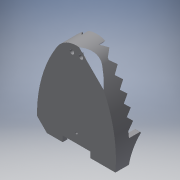
# Autodesk Inventor part: HeadFrame
Saved by Autodesk Inventor 2016 (Build 200138000, 138)
## iProperties
Created: 2017-03-13
Part Number: HeadFrame
Material: Generic
Document SubType Name: Modeling
Designer: Owner
Density: 1 g/cm^3
Appearance: Default
Author: Owner
Autodesk Inventor part; units mm, degrees
sketch "Sketch1" plane through (0, 0, 0) normal (0, 0, 1) x (1, 0, 0)
  line L0 (43.1, 62.15) -> (-43.1, 62.15) projected
  line L1 (43.1, 62.15) -> (-43.1, 62.15)
  line L2 (-43.1, 62.15) -> (-43.1, 176.45)
  line L3 (-43.1, 176.45) -> (43.1, 176.45)
  line L4 (43.1, 176.45) -> (43.1, 62.15)
  arc A0 (43.1, 62.15) -> (21.3882, 150.6616) centre (-96.2036, 74.8977) ccw
  arc A1 (-21.3307, 150.6382) -> (-43.1, 62.15) centre (96.939, 74.6204) ccw
  arc A2 (21.3882, 150.6616) -> (-21.3307, 150.6382) centre (0.0363, 136.9046) ccw
  point P0 (0, 0)
  dimension "d0" = 114.3
  dimension "d1" = 25.4
  constraints: 8 end point, 6 point on circle, 3 centre point, 2 parallel, 2 tangent, 1 horizontal, 1 perpendicular
  measures "d0" distance of L3.end L0.start
  measures "d1" radius of A2
extrude "Extrusion1" add sketch "Sketch1" against normal blind 5 contours L0 L2 A1 A2 A0 L4 | L4 A0 | A1 L2
sketch "Sketch2" plane through (0, 0, -5) normal (0, 0, -1) x (-1, 0, 0)
  arc A0 (-21.3882, 150.6616) -> (-43.1, 62.15) centre (96.2036, 74.8977) ccw projected
  line L0 (-43.1, 62.15) -> (43.1, 62.15) projected
  arc A1 (43.1, 62.15) -> (21.3307, 150.6382) centre (-96.939, 74.6204) ccw projected
  arc A2 (21.3307, 150.6382) -> (-21.3882, 150.6616) centre (-0.0363, 136.9046) ccw projected
  arc A3 (-16.0502, 147.2223) -> (-32.7704, 90.1915) centre (72.1437, 90.3994) ccw
  arc A4 (32.7315, 90.1915) -> (15.989, 147.2048) centre (-72.7133, 90.1915) ccw
  arc A5 (15.989, 147.2048) -> (-16.0502, 147.2223) centre (-0.0363, 136.9046) ccw
  line L1 (-43.1, 62.15) -> (43.1, 62.15) projected
  line L2 (-32.3341, 62.15) -> (32.3159, 62.15)
  line L3 (32.7315, 90.1915) -> (32.7315, 62.15)
  line L4 (32.7315, 62.15) -> (-32.7704, 62.15)
  line L5 (-32.7704, 62.15) -> (-32.7704, 90.1915)
  point P0 (0, 0)
  constraints: 8 end point, 6 point on circle, 3 centre point, 2 point on line, 1 parallel
extrude "Extrusion2" add sketch "Sketch2" along normal blind 10 contours A2 A1 L0 L3 A4 A5 A3 L5 A0
sketch "Sketch3" plane through (-32.7315, 62.15, -5) normal (1, 0, 0) x (0, 0, -1)
  line L0 (0, 0) -> (25, 0)
  line L1 (-5, 0) -> (10, 0) projected
  line L2 (10, 0) -> (10, 25.4)
  arc A0 (25, 0) -> (10, 25.4) centre (-9.2015, -3.0686) ccw
  line L3 (10, 25.4) -> (10, -0.6619)
  line L4 (25, 0) -> (10, 0)
  line L5 (10, 0) -> (10, 25.4)
  point P0 (-5, -62.15)
  dimension "d6" = 25
  dimension "d7" = 25.4
  constraints: 10 end point, 2 collinear, 2 perpendicular, 2 point on circle, 1 centre point, 1 vertical
  measures "d6" distance of L0.start L0.end
  measures "d7" distance of L1.end L2.end
extrude "Extrusion3" add sketch "Sketch3" along normal blind 101.6 and the other way blind 25.4
sketch "Sketch4" plane through (0, 0, -15) normal (0, 0, -1) x (-1, 0, 0)
  line L0 (32.7315, 62.15) -> (32.7315, 90.1915) projected
  arc A0 (32.7315, 90.1915) -> (15.989, 147.2048) centre (-72.7133, 90.1915) ccw projected
  arc A1 (15.989, 147.2048) -> (-16.0502, 147.2223) centre (-0.0363, 136.9046) ccw projected
  arc A2 (-16.0502, 147.2223) -> (-32.7704, 90.1915) centre (72.1437, 90.3994) ccw projected
  line L1 (-32.7704, 90.1915) -> (-32.7704, 62.15) projected
  line L2 (-32.7704, 62.15) -> (32.7315, 62.15) projected
  arc A3 (-21.3882, 150.6616) -> (-43.1087, 87.55) centre (96.2036, 74.8977) ccw projected
  line L3 (-21.3882, 150.6616) -> (-130.3093, 136.9046)
  line L4 (-130.3093, 136.9046) -> (-112.871, 20.9919)
  arc A4 (-21.3882, 150.6616) -> (-43.1, 62.15) centre (96.2036, 74.8977) ccw projected
  line L5 (-43.1, 62.15) -> (-112.871, 20.9919)
  arc A5 (43.0584, 87.55) -> (21.3307, 150.6382) centre (-96.939, 74.6204) ccw projected
  line L6 (21.3307, 150.6382) -> (115.9935, 147.2223)
  line L7 (115.9935, 147.2223) -> (119.9418, 13.6964)
  line L8 (119.9418, 13.6964) -> (43.1, 62.15)
  arc A6 (43.1, 62.15) -> (43.0584, 87.55) centre (-96.939, 74.6204) ccw projected
  point P0 (0, 0)
  constraints: 12 end point, 1 point on circle
extrude "Extrusion4" cut sketch "Sketch4" along normal blind 25.4
sketch "Sketch5" plane through (0, 0, -15) normal (0, 0, -1) x (-1, 0, 0)
  arc A0 (15.989, 147.2048) -> (-16.0502, 147.2223) centre (-0.0363, 136.9046) ccw projected
  line L0 (32.7315, 62.15) -> (32.7315, 90.1915) projected
  arc A1 (32.7315, 90.1915) -> (15.989, 147.2048) centre (-72.7133, 90.1915) ccw projected
  arc A2 (15.989, 147.2048) -> (-16.0502, 147.2223) centre (-0.0363, 136.9046) ccw projected
  arc A3 (-16.0502, 147.2223) -> (-32.7704, 90.1915) centre (72.1437, 90.3994) ccw projected
  line L1 (-32.7704, 90.1915) -> (-32.7704, 62.15) projected
  line L2 (-32.7704, 62.15) -> (32.7315, 62.15) projected
  arc A4 (43.0584, 87.55) -> (21.3307, 150.6382) centre (-96.939, 74.6204) ccw projected
  arc A5 (21.3307, 150.6382) -> (-21.3882, 150.6616) centre (-0.0363, 136.9046) ccw projected
  arc A6 (-21.3882, 150.6616) -> (-43.1087, 87.55) centre (96.2036, 74.8977) ccw projected
  line L3 (-0.0224, 162.3046) -> (-0.0224, 87.55)
  line L4 (-0.0224, 87.55) -> (-0.0224, 100.25)
  line L5 (-0.0224, 100.25) -> (41.2983, 100.25)
  line L6 (41.2983, 100.25) -> (-41.3655, 100.25)
  line L7 (41.2983, 111.68) -> (-41.3655, 111.68)
  line L8 (41.2983, 123.11) -> (-41.3655, 123.11)
  line L9 (41.2983, 134.54) -> (-41.3655, 134.54)
  line L10 (41.2983, 145.97) -> (-41.3655, 145.97)
  line L11 (41.2983, 157.4) -> (-41.3655, 157.4)
  point P0 (0, 0)
  dimension "d15" = 12.7
  dimension "d18" = 11.43
  constraints: 18 end point, 3 point on circle, 2 point on line, 2 vertical, 1 perpendicular, 15 other
  measures "d15" distance of L3.end L4.end
  measures "d18" distance of L5.end L7.start
ref_plane "Work Plane1" through (24.2818, 145.97, -15) normal (0.8613, 0.5081, 0) x (-0.5081, 0.8613, 0)
ref_plane "Work Plane2" through (30.3302, 134.54, -15) normal (0.9046, 0.4264, 0) x (-0.4264, 0.9046, 0)
ref_plane "Work Plane3" through (35.1112, 123.11, -15) normal (0.9387, 0.3447, 0) x (-0.3447, 0.9387, 0)
ref_plane "Work Plane4" through (38.7596, 111.68, -15) normal (0.9648, 0.2629, 0) x (-0.2629, 0.9648, 0)
ref_plane "Work Plane5" through (41.3655, 100.25, -15) normal (0.9834, 0.1812, 0) x (-0.1812, 0.9834, 0)
ref_plane "Work Plane6" through (15.0396, 157.4, -15) normal (0.5907, 0.8069, 0) x (-0.8069, 0.5907, 0)
sketch "Sketch6" plane through (15.0396, 157.4, -15) normal (0.5907, 0.8069, 0) x (-0.8069, 0.5907, 0)
  line L0 (0, 0) -> (-6.35, 0)
  line L1 (-9.103, 0) -> (25.4, 0) projected
  line L2 (-6.35, 0) -> (6.35, 0)
  line L3 (0, 0) -> (0, -6.35)
  line L4 (0, -6.35) -> (6.35, 0)
  line L5 (0, -6.35) -> (-6.35, 0)
  point P0 (-80.8377, 15)
  point P1 (25.3533, 0)
  dimension "d23" = 6.35
  dimension "d24" = 12.7
  dimension "d25" = 6.35
  constraints: 10 end point, 2 point on line, 1 vertical
  measures "d23" distance of L0.start L0.end
  measures "d24" distance of L0.end L2.end
  measures "d25" distance of L0.start L3.end
sketch "Sketch7" plane through (24.2818, 145.97, -15) normal (0.8613, 0.5081, 0) x (-0.5081, 0.8613, 0)
  line L0 (0, 0) -> (-6.35, 0)
  line L1 (-9.103, 0) -> (25.4, 0)
  line L2 (-6.35, 0) -> (6.35, 0)
  line L3 (0, 0) -> (0, -6.35)
  line L4 (0, -6.35) -> (6.35, 0)
  line L5 (0, -6.35) -> (-6.35, 0)
  point P0 (-113.389, 15)
  point P1 (25.3533, 0)
  dimension "d26" = 6.35
  dimension "d27" = 12.7
  dimension "d28" = 6.35
  constraints: 12 end point, 2 point on line, 1 vertical
  measures "d26" distance of L0.start L0.end
  measures "d27" distance of L0.end L2.end
  measures "d28" distance of L0.start L3.end
sketch "Sketch8" plane through (30.3302, 134.54, -15) normal (0.9046, 0.4264, 0) x (-0.4264, 0.9046, 0)
  line L0 (0, 0) -> (-6.35, 0)
  line L1 (-9.103, 0) -> (25.4, 0)
  line L2 (-6.35, 0) -> (6.35, 0)
  line L3 (0, 0) -> (0, -6.35)
  line L4 (0, -6.35) -> (6.35, 0)
  line L5 (0, -6.35) -> (-6.35, 0)
  point P0 (-108.7666, 15)
  point P1 (25.3533, 0)
  dimension "d29" = 6.35
  dimension "d30" = 12.7
  dimension "d31" = 6.35
  constraints: 12 end point, 2 point on line, 1 vertical
  measures "d29" distance of L0.start L0.end
  measures "d30" distance of L0.end L2.end
  measures "d31" distance of L0.start L3.end
sketch "Sketch9" plane through (35.1112, 123.11, -15) normal (0.9387, 0.3447, 0) x (-0.3447, 0.9387, 0)
  line L0 (0, 0) -> (-6.35, 0)
  line L1 (-9.103, 0) -> (25.4, 0)
  line L2 (-6.35, 0) -> (6.35, 0)
  line L3 (0, 0) -> (0, -6.35)
  line L4 (0, -6.35) -> (6.35, 0)
  line L5 (0, -6.35) -> (-6.35, 0)
  point P0 (-103.4657, 15)
  point P1 (25.3533, 0)
  dimension "d32" = 6.35
  dimension "d33" = 12.7
  dimension "d34" = 6.35
  constraints: 12 end point, 2 point on line, 1 vertical
  measures "d32" distance of L0.start L0.end
  measures "d33" distance of L0.end L2.end
  measures "d34" distance of L0.start L3.end
sketch "Sketch10" plane through (38.7596, 111.68, -15) normal (0.9648, 0.2629, 0) x (-0.2629, 0.9648, 0)
  line L0 (0, 0) -> (-6.35, 0)
  line L1 (-9.103, 0) -> (25.4, 0)
  line L2 (-6.35, 0) -> (6.35, 0)
  line L3 (0, 0) -> (0, -6.35)
  line L4 (0, -6.35) -> (6.35, 0)
  line L5 (0, -6.35) -> (-6.35, 0)
  point P0 (-97.5584, 15)
  point P1 (25.3533, 0)
  dimension "d35" = 6.35
  dimension "d36" = 12.7
  dimension "d37" = 6.35
  constraints: 12 end point, 2 point on line, 1 vertical
  measures "d35" distance of L0.start L0.end
  measures "d36" distance of L0.end L2.end
  measures "d37" distance of L0.start L3.end
sketch "Sketch11" plane through (41.3655, 100.25, -15) normal (0.9834, 0.1812, 0) x (-0.1812, 0.9834, 0)
  line L0 (0, 0) -> (-6.35, 0)
  line L1 (-9.103, 0) -> (25.4, 0)
  line L2 (-6.35, 0) -> (6.35, 0)
  line L3 (0, 0) -> (0, -6.35)
  line L4 (0, -6.35) -> (6.35, 0)
  line L5 (0, -6.35) -> (-6.35, 0)
  point P0 (-91.0929, 15)
  point P1 (25.3533, 0)
  dimension "d38" = 6.35
  dimension "d39" = 12.7
  dimension "d40" = 6.35
  constraints: 12 end point, 2 point on line, 1 vertical
  measures "d38" distance of L0.start L0.end
  measures "d39" distance of L0.end L2.end
  measures "d40" distance of L0.start L3.end
extrude "Extrusion5" add sketch "Sketch7" against normal blind 25.4
extrude "Extrusion6" add sketch "Sketch6" against normal blind 25.4
extrude "Extrusion7" add sketch "Sketch8" against normal blind 25.4
extrude "Extrusion8" add sketch "Sketch9" against normal blind 25.4
extrude "Extrusion9" add sketch "Sketch10" against normal blind 25.4
extrude "Extrusion10" add sketch "Sketch11" against normal blind 25.4
ref_plane "Work Plane7" through (-14.967, 157.4, -15) normal (-0.5907, 0.8069, 0) x (-0.8069, -0.5907, 0)
ref_plane "Work Plane8" through (-24.2042, 145.97, -15) normal (-0.8617, 0.5075, 0) x (-0.5075, -0.8617, 0)
ref_plane "Work Plane9" through (-30.2462, 134.54, -15) normal (-0.9046, 0.4262, 0) x (-0.4262, -0.9046, 0)
ref_plane "Work Plane10" through (-35.0276, 123.11, -15) normal (-0.9386, 0.3449, 0) x (-0.3449, -0.9386, 0)
ref_plane "Work Plane11" through (-38.6819, 111.68, -15) normal (-0.9646, 0.2636, 0) x (-0.2636, -0.9646, 0)
ref_plane "Work Plane12" through (-41.2983, 100.25, -15) normal (-0.9832, 0.1823, 0) x (-0.1823, -0.9832, 0)
sketch "Sketch13" plane through (-14.967, 157.4, -15) normal (-0.5907, 0.8069, 0) x (-0.8069, -0.5907, 0)
  line L0 (0, 0) -> (-6.35, 0)
  line L1 (6.8467, 0) -> (-15.2019, 0) projected
  line L2 (-6.35, 0) -> (6.35, 0)
  line L3 (0, 0) -> (0, -6.35)
  line L4 (0, -6.35) -> (-6.35, 0)
  line L5 (0, -6.35) -> (6.35, 0)
  point P0 (80.8962, 15)
  dimension "d56" = 6.35
  dimension "d57" = 12.7
  dimension "d58" = 6.35
  constraints: 10 end point, 2 point on line, 1 vertical
  measures "d56" distance of L0.start L0.end
  measures "d57" distance of L0.end L2.end
  measures "d58" distance of L0.start L3.end
sketch "Sketch14" plane through (-24.2042, 145.97, -15) normal (-0.8617, 0.5075, 0) x (-0.5075, -0.8617, 0)
  line L0 (0, 0) -> (-6.35, 0)
  line L1 (6.8467, 0) -> (-15.2019, 0)
  line L2 (-6.35, 0) -> (6.35, 0)
  line L3 (0, 0) -> (0, -6.35)
  line L4 (0, -6.35) -> (-6.35, 0)
  line L5 (0, -6.35) -> (6.35, 0)
  point P0 (113.4928, 15)
  dimension "d59" = 6.35
  dimension "d60" = 12.7
  dimension "d61" = 6.35
  constraints: 12 end point, 2 point on line, 1 vertical
  measures "d59" distance of L0.start L0.end
  measures "d60" distance of L0.end L2.end
  measures "d61" distance of L0.start L3.end
sketch "Sketch15" plane through (-30.2462, 134.54, -15) normal (-0.9046, 0.4262, 0) x (-0.4262, -0.9046, 0)
  line L0 (0, 0) -> (-6.35, 0)
  line L1 (6.8467, 0) -> (-15.2019, 0)
  line L2 (-6.35, 0) -> (6.35, 0)
  line L3 (0, 0) -> (0, -6.35)
  line L4 (0, -6.35) -> (-6.35, 0)
  line L5 (0, -6.35) -> (6.35, 0)
  point P0 (108.8187, 15)
  dimension "d62" = 6.35
  dimension "d63" = 12.7
  dimension "d64" = 6.35
  constraints: 12 end point, 2 point on line, 1 vertical
  measures "d62" distance of L0.start L0.end
  measures "d63" distance of L0.end L2.end
  measures "d64" distance of L0.start L3.end
sketch "Sketch16" plane through (-35.0276, 123.11, -15) normal (-0.9386, 0.3449, 0) x (-0.3449, -0.9386, 0)
  line L0 (0, 0) -> (-6.35, 0)
  line L1 (6.8467, 0) -> (-15.2019, 0)
  line L2 (-6.35, 0) -> (6.35, 0)
  line L3 (0, 0) -> (0, -6.35)
  line L4 (0, -6.35) -> (-6.35, 0)
  line L5 (0, -6.35) -> (6.35, 0)
  point P0 (103.4754, 15)
  dimension "d65" = 6.35
  dimension "d66" = 12.7
  dimension "d67" = 6.35
  constraints: 12 end point, 2 point on line, 1 vertical
  measures "d65" distance of L0.start L0.end
  measures "d66" distance of L0.end L2.end
  measures "d67" distance of L0.start L3.end
sketch "Sketch17" plane through (-38.6819, 111.68, -15) normal (-0.9646, 0.2636, 0) x (-0.2636, -0.9646, 0)
  line L0 (0, 0) -> (-6.35, 0)
  line L1 (6.8467, 0) -> (-15.2019, 0)
  line L2 (-6.35, 0) -> (6.35, 0)
  line L3 (0, 0) -> (0, -6.35)
  line L4 (0, -6.35) -> (-6.35, 0)
  line L5 (0, -6.35) -> (6.35, 0)
  point P0 (97.5339, 15)
  dimension "d68" = 6.35
  dimension "d69" = 12.7
  dimension "d70" = 6.35
  constraints: 12 end point, 2 point on line, 1 vertical
  measures "d68" distance of L0.start L0.end
  measures "d69" distance of L0.end L2.end
  measures "d70" distance of L0.start L3.end
sketch "Sketch18" plane through (-41.2983, 100.25, -15) normal (-0.9832, 0.1823, 0) x (-0.1823, -0.9832, 0)
  line L0 (0, 0) -> (-6.35, 0)
  line L1 (6.8467, 0) -> (-15.2019, 0)
  line L2 (-6.35, 0) -> (6.35, 0)
  line L3 (0, 0) -> (0, -6.35)
  line L4 (0, -6.35) -> (-6.35, 0)
  line L5 (0, -6.35) -> (6.35, 0)
  point P0 (91.0417, 15)
  dimension "d71" = 6.35
  dimension "d72" = 12.7
  dimension "d73" = 6.35
  constraints: 12 end point, 2 point on line, 1 vertical
  measures "d71" distance of L0.start L0.end
  measures "d72" distance of L0.end L2.end
  measures "d73" distance of L0.start L3.end
extrude "Extrusion11" add sketch "Sketch13" against normal blind 25.4
extrude "Extrusion12" add sketch "Sketch14" against normal blind 25.4
extrude "Extrusion13" add sketch "Sketch15" against normal blind 25.4
extrude "Extrusion14" add sketch "Sketch16" against normal blind 25.4
extrude "Extrusion15" add sketch "Sketch17" against normal blind 25.4
extrude "Extrusion16" add sketch "Sketch18" against normal blind 25.4
sketch "Sketch19" plane through (0, 0, -5) normal (0, 0, -1) x (-1, 0, 0)
  line L0 (32.7315, 62.15) -> (32.7315, 90.1915) projected
  arc A0 (32.7315, 90.1915) -> (15.989, 147.2048) centre (-72.7133, 90.1915) ccw projected
  arc A1 (15.989, 147.2048) -> (-16.0502, 147.2223) centre (-0.0363, 136.9046) ccw projected
  arc A2 (-16.0502, 147.2223) -> (-32.7704, 90.1915) centre (72.1437, 90.3994) ccw projected
  line L1 (-32.7704, 90.1915) -> (-32.7704, 62.15) projected
  line L2 (-32.7704, 62.15) -> (32.7315, 62.15) projected
  point P0 (0, 0)
extrude "Extrusion17" cut sketch "Sketch19" along normal blind 25.4
sketch "Sketch20" plane through (0, 0, 0) normal (0, 0, 1) x (1, 0, 0)
  arc A0 (21.3882, 150.6616) -> (-21.3307, 150.6382) centre (0.0363, 136.9046) ccw projected
  arc A1 (-21.3307, 150.6382) -> (-43.1, 62.15) centre (96.939, 74.6204) ccw projected
  arc A2 (43.1, 62.15) -> (21.3882, 150.6616) centre (-96.2036, 74.8977) ccw projected
  line L0 (43.1, 62.15) -> (-43.1, 62.15) projected
  line L1 (-43.1, 62.15) -> (-82.9199, 62.15)
  line L2 (-82.9199, 62.15) -> (-48.8812, 239.8541)
  line L3 (-48.8812, 239.8541) -> (69.4627, 239.8541)
  line L4 (69.4627, 239.8541) -> (43.1, 62.15)
  point P0 (0, 0)
  constraints: 8 end point, 1 horizontal, 1 parallel
extrude "Extrusion18" cut sketch "Sketch20" against normal blind 101.6 contours A0 A1 L1 L2 L3 L4 A2
sketch "Sketch21" plane through (32.7704, 62.15, -5) normal (-1, 0, 0) x (0, 0, 1)
  arc A0 (-10, 25.4) -> (-25, 0) centre (9.2015, -3.0686) ccw projected
  line L0 (-10, 25.4) -> (-10, 0)
  line L1 (-25, 0) -> (0, 0) projected
  line L2 (-50.1881, 0) -> (-12.0881, 0)
  line L3 (5, 0) -> (-25, 0) projected
  point P0 (5, -62.15)
  constraints: 4 end point, 1 horizontal, 1 point on line, 1 vertical, 3 other
extrude "Extrusion19" cut sketch "Sketch21" along normal mid plane 826363.6
sketch "Sketch22" plane through (32.7704, 62.15, -5) normal (-1, 0, 0) x (0, 0, 1)
  spline S0 degree 3 poles (-25, 25.4) (-23.1271, 24.1368) (-21.4071, 22.7039) (-18.3633, 19.6512) (-16.9356, 17.9273) (-14.4203, 14.175) (-13.3326, 12.1465) (-11.5878, 7.9192) (-10.9291, 5.7167) (-10.2695, 2.3351) (-10.1043, 1.1624) (-10, 0) knots 12.377494 12.377494 12.377494 12.377494 13.025034 13.025034 13.671951 13.671951 14.318868 14.318868 14.965786 14.965786 15.308147 15.308147 15.308147 15.308147
  line L0 (-25, 25.4) -> (-10, 25.4)
  line L1 (-10, 0) -> (-10, 28.0415) projected
  line L2 (-10, 0) -> (-10, 25.4)
  point P0 (5, -62.15)
  constraints: 4 end point, 1 horizontal, 1 perpendicular, 1 point on line, 4 other
extrude "Extrusion20" add sketch "Sketch22" along normal blind 101.6 and the other way blind 25.4
sketch "Sketch23" plane through (0, 0, -5) normal (0, 0, -1) x (-1, 0, 0)
  arc A0 (-16.0278, 147.2048) -> (-32.7704, 90.1915) centre (72.6745, 90.1915) ccw
  line L0 (-32.7704, 62.15) -> (-32.7704, 90.1915)
  line L1 (43.0611, 62.15) -> (-43.1389, 62.15)
  line L2 (32.7315, 90.1915) -> (32.7315, 62.15)
  arc A1 (32.7315, 90.1915) -> (16.0114, 147.2223) centre (-72.1825, 90.3994) ccw
  arc A2 (16.0114, 147.2223) -> (-16.0278, 147.2048) centre (-0.0026, 136.9046) ccw
  arc A3 (-21.3696, 150.6382) -> (-43.1389, 62.15) centre (96.9002, 74.6204) ccw
  arc A4 (43.0611, 62.15) -> (21.3494, 150.6616) centre (-96.2425, 74.8977) ccw
  line L3 (32.7315, 62.15) -> (32.7315, 90.1915) projected
  arc A5 (32.7315, 90.1915) -> (15.989, 147.2048) centre (-72.7133, 90.1915) ccw projected
  arc A6 (15.989, 147.2048) -> (-16.0502, 147.2223) centre (-0.0363, 136.9046) ccw projected
  arc A7 (-16.0502, 147.2223) -> (-32.7704, 90.1915) centre (72.1437, 90.3994) ccw projected
  line L4 (-32.7704, 90.1915) -> (-32.7704, 62.15) projected
  line L5 (-32.7704, 62.15) -> (32.7315, 62.15) projected
  arc A8 (15.989, 147.2048) -> (-16.0502, 147.2223) centre (-0.0363, 136.9046) ccw projected
  arc A9 (-16.0502, 147.2223) -> (-32.7704, 90.1915) centre (72.1437, 90.3994) ccw projected
  point P0 (0, 0)
  constraints: 10 point on circle, 6 end point, 5 centre point, 2 vertical, 1 horizontal, 20 other
extrude "Extrusion21" cut sketch "Sketch23" along normal blind 101.6
sketch "Sketch24" plane through (0, 0, 0) normal (0, 0, 1) x (1, 0, 0)
  arc A0 (43.1, 62.15) -> (21.3882, 150.6616) centre (-96.2036, 74.8977) ccw projected
  arc A1 (21.3882, 150.6616) -> (-21.3307, 150.6382) centre (0.0363, 136.9046) ccw projected
  arc A2 (-21.3307, 150.6382) -> (-43.1, 62.15) centre (96.939, 74.6204) ccw projected
  line L0 (-43.1, 62.15) -> (43.1, 62.15) projected
  line L1 (-43.1, 62.15) -> (-100.8319, 32.0272)
  line L2 (-100.8319, 32.0272) -> (-90.1051, 110.1795)
  line L3 (-90.1051, 110.1795) -> (-39.083, 110.1795)
  line L4 (39.1596, 110.1795) -> (129.641, 110.1795)
  line L5 (129.641, 110.1795) -> (126.8827, 23.1392)
  line L6 (126.8827, 23.1392) -> (43.1, 62.15)
  point P0 (0, 0)
  constraints: 12 end point, 2 point on circle, 2 point on line, 1 horizontal
extrude "Extrusion22" cut sketch "Sketch24" against normal blind 101.6 contours A0 L4 L5 L6 | L1 L2 L3 A2
sketch "Sketch25" plane through (0, 0, 0) normal (0, 0, 1) x (1, 0, 0)
  line L0 (32.7704, 62.15) -> (-32.7315, 62.15) projected
  line L1 (0.0194, 62.15) -> (-15.2206, 62.15)
  line L2 (-15.2206, 62.15) -> (15.2594, 62.15)
  line L3 (15.2594, 62.15) -> (15.2594, 68.5)
  line L4 (15.2594, 68.5) -> (-15.2206, 68.5)
  line L5 (-15.2206, 68.5) -> (-15.2206, 62.15)
  point P0 (0, 0)
  dimension "d100" = 15.24
  dimension "d101" = 30.48
  dimension "d102" = 6.35
  constraints: 10 end point, 3 perpendicular, 2 point on line, 1 midpoint
  measures "d100" distance of L1.start L1.end
  measures "d101" distance of L1.end L2.end
  measures "d102" distance of L2.end L3.end
extrude "Extrusion23" cut sketch "Sketch25" against normal blind 101.6
sketch "Sketch26" plane through (0, 0, -5) normal (0, 0, -1) x (-1, 0, 0)
  line L0 (-15.2594, 62.15) -> (-15.2594, 68.5) projected
  line L1 (-15.2594, 68.5) -> (15.2206, 68.5) projected
  line L2 (15.2206, 68.5) -> (15.2206, 62.15) projected
  line L3 (15.2206, 62.15) -> (32.7315, 62.15) projected
  line L4 (32.7315, 62.15) -> (32.7315, 90.1915) projected
  arc A0 (32.7315, 90.1915) -> (15.989, 147.2048) centre (-72.7133, 90.1915) ccw projected
  arc A1 (15.989, 147.2048) -> (-16.0502, 147.2223) centre (-0.0363, 136.9046) ccw projected
  arc A2 (-16.0502, 147.2223) -> (-32.7704, 90.1915) centre (72.1437, 90.3994) ccw projected
  line L5 (-32.7704, 90.1915) -> (-32.7704, 62.15) projected
  line L6 (-32.7704, 62.15) -> (-15.2594, 62.15) projected
  line L7 (-17.5429, 50.9368) -> (-17.5429, 58.2393)
  line L8 (-17.5429, 58.2393) -> (17.5091, 58.2393)
  line L9 (17.5091, 58.2393) -> (17.5091, 50.9368)
  line L10 (17.5091, 50.9368) -> (37.6467, 50.9368)
  line L11 (37.6467, 50.9368) -> (37.6467, 83.1845)
  arc A3 (37.6467, 83.1845) -> (18.3928, 148.7499) centre (-83.6149, 83.1845) ccw
  arc A4 (18.3928, 148.7499) -> (-18.4523, 148.77) centre (-0.0363, 136.9046) ccw
  arc A5 (-18.4523, 148.77) -> (-37.6805, 83.1845) centre (82.9706, 83.4237) ccw
  line L12 (-37.6805, 83.1845) -> (-37.6805, 50.9368)
  line L13 (-37.6805, 50.9368) -> (-17.5429, 50.9368)
  point P0 (0, 0)
  constraints: 14 end point, 6 point on circle, 3 centre point
extrude "Extrusion24" cut sketch "Sketch26" along normal blind 25.4
sketch "Sketch27" plane through (0, 0, -15) normal (0, 0, -1) x (-1, 0, 0)
  arc A0 (7.2247, 157.5738) -> (-7.2972, 157.5738) centre (-0.0363, 136.9046) ccw projected
  line L0 (7.2247, 157.5738) -> (9.3668, 160.5) projected
  arc A1 (9.3668, 160.5) -> (-9.4393, 160.5) centre (-0.0363, 136.9046) ccw projected
  line L1 (-9.4393, 160.5) -> (-7.2972, 157.5738) projected
  point P0 (0, 0)
extrude "Extrusion25" add sketch "Sketch27" along normal blind 7.5
fillet "Fillet1" radius 1 2 edges at (40.3594, 87.55, -30) (-40.3132, 87.55, -30)
sketch "Sketch28" plane through (0, 0, 0) normal (0, 0, 1) x (1, 0, 0)
  arc A0 (7.2972, 157.5738) -> (-7.2247, 157.5738) centre (0.0363, 136.9046) ccw projected
  line L0 (0.0363, 136.9046) -> (0.0363, 158.8121)
  line L1 (0.0363, 158.8121) -> (0.0363, 153.8121)
  line L2 (0.0363, 153.8121) -> (5.0363, 153.8121)
  line L3 (5.0363, 153.8121) -> (-4.9637, 153.8121)
  circle A1 centre (5.0363, 153.8121) radius 2.4125
  circle A2 centre (-4.9637, 153.8121) radius 2.4125
  point P0 (0, 0)
  dimension "d110" = 5
  dimension "d111" = 5
  dimension "d112" = 10
  dimension "d113" = 4.825
  dimension "d114" = 4.825
  constraints: 8 end point, 2 centre point, 2 coincident, 2 point on line, 1 perpendicular, 1 point on circle, 1 vertical
  measures "d110" distance of L0.end L1.end
  measures "d111" distance of L1.end L2.end
  measures "d112" distance of L2.end L3.end
  measures "d113" diameter of A1
  measures "d114" diameter of A2
extrude "Extrusion26" cut sketch "Sketch28" against normal blind 25.4
sketch "Sketch29" plane through (0, 0, 0) normal (0, 0, 1) x (1, 0, 0)
  circle A0 centre (0.0258, 78.5) radius 1.5
  circle A1 centre (0.0258, 78.5) radius 1.25
  point P0 (0, 0)
  dimension "d117" = 2.5
  constraints: 2 centre point, 1 coincident, 2 other
  measures "d117" diameter of A1
extrude "Extrusion27" cut sketch "Sketch29" against normal blind 25.4 contours A1
body "Solid1"
